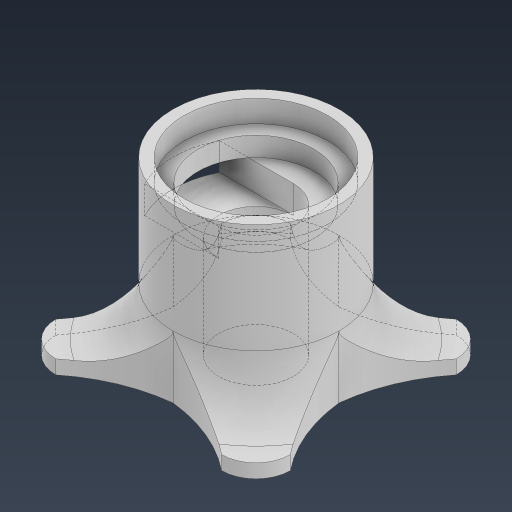
# Autodesk Inventor part: Base
Saved by Autodesk Inventor 2024 (Build 280153000, 153)
## iProperties
Created: 2025-08-29
Part Number: Base
Material: Generic
Document SubType Name: Modeling
Designer: Piter
Density: 1 g/cm^3
Appearance: Default
Author: Piter
Autodesk Inventor part; units mm, degrees
ref_plane "YZ Plane" through (0, 0, 0) normal (1, 0, 0) x (0, 1, 0)
ref_plane "XZ Plane" through (0, 0, 0) normal (0, 1, 0) x (-1, 0, 0)
ref_plane "XY Plane" through (0, 0, 0) normal (0, 0, 1) x (1, 0, 0)
sketch "Sketch1" plane through (0, 0, 0) normal (0, 1, 0) x (-1, 0, 0)
  circle A0 centre (0, 0) radius 26.05
  circle A1 centre (0, 0) radius 21
  circle A2 centre (0, 0) radius 30
  dimension "d0" = 52.1
  dimension "d1" = 60
  dimension "d6" = 42
  constraints: 3 centre point, 3 coincident
  measures "d0" diameter of A0
  measures "d1" diameter of A2
  measures "d6" diameter of A1
extrude "Extrusion1" add sketch "Sketch1" along normal blind 17 contours A2
extrude "Extrusion2" add sketch "Sketch1" along normal blind 9 contours A0
extrude "Extrusion3" add sketch "Sketch1" along normal blind 2 contours A1
sketch "Sketch2" plane through (0, 2, 0) normal (0, 1, 0) x (1, 0, 0)
  circle A0 centre (0, 0) radius 13.5
  dimension "d9" = 27
  constraints: 1 centre point, 1 coincident
  measures "d9" diameter of A0
extrude "Extrusion4" cut sketch "Sketch2" against normal through all
sketch "Sketch3" plane through (0, 0, 0) normal (0, -1, 0) x (1, 0, 0)
  circle A0 centre (0, 0) radius 30 projected
  circle A1 centre (0, 0) radius 13.5 projected
  circle A2 centre (0, 0) radius 30 projected
extrude "Main_height" add sketch "Sketch3" along normal blind 40
sketch "Sketch4" plane through (0, 0, 0) normal (1, 0, 0) x (0, 1, 0)
  line L0 (2, 13.5) -> (2, -13.5) projected
  line L1 (2, -13.5) -> (-40, -13.5) projected
  line L2 (2, 13.5) -> (-8, 13.5)
  line L3 (-8, 13.5) -> (-8, -13.5)
  line L4 (-8, -13.5) -> (2, -13.5)
  line L5 (2, -13.5) -> (2, 13.5)
  point P0 (0, 0)
  constraints: 8 end point, 2 parallel, 1 horizontal, 1 perpendicular, 1 point on line
extrude "Extrusion6" cut sketch "Sketch4" against normal through all
sketch "Sketch5" plane through (0, -40, 0) normal (0, -1, 0) x (1, 0, 0)
  line L0 (-30, -30) -> (30, -30)
  line L1 (30, -30) -> (30, 30)
  line L2 (30, 30) -> (-30, 30)
  line L3 (-30, 30) -> (-30, -30)
  line L4 (-30, -30) -> (30, 30) construction
  line L5 (30, -30) -> (-30, 30) construction
  circle A0 centre (0, 0) radius 30 projected
  circle A1 centre (-30, 30) radius 12.4264
  arc A2 (-30, 42.4264) -> (0, 30) centre (6.3083, 87.6559) ccw
  arc A3 (-30, 0) -> (-42.4264, 30) centre (-87.6559, -6.3083) ccw
  line L6 (0, 30) -> (0, -30) construction
  line L7 (-30, 0) -> (31, 0) construction
  circle A4 centre (30, 30) radius 12.4264
  arc A5 (0, 30) -> (30, 42.4264) centre (-6.3083, 87.6559) ccw
  arc A6 (42.4264, 30) -> (30, 0) centre (87.6559, -6.3083) ccw
  circle A7 centre (-30, -30) radius 12.4264
  arc A8 (0, -30) -> (-30, -42.4264) centre (6.3083, -87.6559) ccw
  arc A9 (-42.4264, -30) -> (-30, 0) centre (-87.6559, 6.3083) ccw
  circle A10 centre (30, -30) radius 12.4264
  arc A11 (30, -42.4264) -> (0, -30) centre (-6.3083, -87.6559) ccw
  arc A12 (30, 0) -> (42.4264, -30) centre (87.6559, 6.3083) ccw
  circle A13 centre (0, 0) radius 13.5 projected
  point P0 (18.7934, 35.3692)
  point P1 (35.3692, 18.7934)
  dimension "d16" = 60
  dimension "d17" = 60
  dimension "d18" = 58
  dimension "d19" = 58
  constraints: 27 point on circle, 16 end point, 16 symmetric about line, 12 centre point, 5 midpoint, 2 parallel, 2 perpendicular, 1 coincident, 1 horizontal, 9 other
  measures "d16" distance of L2.end L1.end
  measures "d17" distance of L1.end L0.end
  measures "d18" radius of A2
  measures "d19" radius of A3
extrude "Extrusion7" add sketch "Sketch5" along normal blind 5 contours L3 A7 L0 | L0 A7 A8 A9 L3 | A7 A0 L0 | L0 A8 A7 | A7 A9 L3 | L3 A0 A7 | A0 A10 L0 | A0 | L0 A10 A11 | A3 A1 L3 | L3 A1 A0 | A10 L1 L0 | L0 L1 A10 A12 A11 | A0 L1 A10 | A1 A3 A2 L2 L3 | L3 L2 A1 | A1 L2 A0 | A12 A10 L1 | A0 A4 L1 | L1 A4 A6 | A5 A4 L2 | L2 A4 A0 | L2 A1 A2 | A4 L2 L1 | L1 L2 A4 A5 A6
fillet "Fillet1" radius 17.5 4 edges at (21.2132, -40, -21.2132) (-21.2132, -40, -21.2132) (-21.2132, -40, 21.2132) (21.2132, -40, 21.2132)
body "Solid1"
